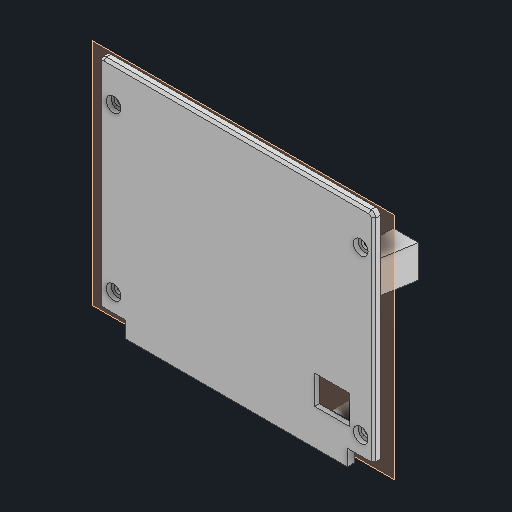
# Autodesk Inventor part: BP_BackCover
Saved by Autodesk Inventor 2026.1 (Build 301233020, 233B)
## iProperties
Created: 2025-09-13
Part Number: BP_BackCover
Material: Generic
Document SubType Name: Modeling
Designer: atrus
Density: 1 g/cm^3
Appearance: Default
Author: atrus
Autodesk Inventor part; units mm, degrees
ref_plane "YZ Plane" through (0, 0, 0) normal (1, 0, 0) x (0, 1, 0)
ref_plane "XZ Plane" through (0, 0, 0) normal (0, 1, 0) x (-1, 0, 0)
ref_plane "XY Plane" through (0, 0, 0) normal (0, 0, 1) x (1, 0, 0)
ref_plane "Work Plane1" through (0, 0, -0.1) normal (0, 0, 1) x (1, 0, 0)
sketch "Sketch1" plane through (0, 0, -0.1) normal (0, 0, 1) x (1, 0, 0)
  circle A0 centre (-111.199, -72) radius 2
  circle A1 centre (-5.483, -2.5) radius 2
  circle A2 centre (-111.199, -2.5) radius 2
  line L0 (-105.066, 0.2) -> (-96.966, 0.2)
  line L1 (-10.366, -5.012) -> (0, -5.012)
  line L2 (0, -5.012) -> (0, 5.5)
  line L3 (-9, 5.5) -> (0, 5.5)
  line L4 (-9, 5.5) -> (-9, 7.2)
  spline S0 degree 3 poles (-11.0328, 9.2) (-10.764, 9.2) (-10.4976, 9.1476) (-10.0026, 8.9441) (-9.7782, 8.7957) (-9.4033, 8.4236) (-9.2552, 8.2048) (-9.0524, 7.7216) (-9, 7.4622) (-9, 7.2) knots 0 0 0 0 0.253656 0.253656 0.505123 0.505123 0.752333 0.752333 1 1 1 1
  line L5 (-106.2992, 9.2) -> (-11.0328, 9.2)
  spline S1 degree 3 poles (-108.332, 7.2) (-108.332, 7.4565) (-108.2819, 7.7103) (-108.0866, 8.187) (-107.9426, 8.4048) (-107.577, 8.7772) (-107.3577, 8.9271) (-106.9875, 9.0869) (-106.8536, 9.1291) (-106.5792, 9.1857) (-106.4394, 9.2) (-106.2992, 9.2) knots 0 0 0 0 0.242386 0.242386 0.486827 0.486827 0.735395 0.735395 0.867613 0.867613 1 1 1 1
  line L6 (-108.332, 5.5) -> (-108.332, 7.2)
  line L7 (-117.332, 5.5) -> (-108.332, 5.5)
  line L8 (-117.332, -80) -> (-117.332, 5.5)
  line L9 (-105.066, -80) -> (-117.332, -80)
  line L10 (-105.066, -80) -> (-105.066, 0.2)
  circle A3 centre (-5.483, -72) radius 2
  line L11 (0, -19.352) -> (-10.366, -19.352)
  line L12 (-10.966, -79.0494) -> (-10.966, -80)
  line L13 (0, -80) -> (-10.966, -80)
  line L14 (0, -19.352) -> (0, -80)
  line L15 (0, -19.352) -> (0, -5.012)
  line L16 (-10.366, 2) -> (-10.366, -5.012)
  line L17 (-96.966, 0.2) -> (-96.966, 2)
  arc A4 (-93.166, 5.8) -> (-96.966, 2) centre (-93.166, 2) ccw
  line L18 (-93.166, 5.8) -> (-14.166, 5.8)
  arc A5 (-10.366, 2) -> (-14.166, 5.8) centre (-14.166, 2) ccw
  line L19 (-10.366, -19.352) -> (-10.366, -77)
  arc A6 (-10.966, -79.0494) -> (-10.366, -77) centre (-14.166, -77) ccw
  line L20 (-10.366, -19.352) -> (-10.366, -5.012)
  line L21 (-105.066, -80) -> (-104.866, -80)
  line L22 (-106.132, -86.7) -> (-11.166, -86.7)
  line L23 (-11.166, -86.7) -> (-11.166, -80)
  line L24 (-11.166, -80) -> (-10.966, -80)
  line L25 (-10.366, -73) -> (-105.066, -73)
  circle A7 centre (-111.199, -72) radius 2
  circle A8 centre (-5.483, -2.5) radius 2
  circle A9 centre (-111.199, -2.5) radius 2
  line L26 (-10.366, 2) -> (-10.366, -5.012)
  line L27 (-10.366, -5.012) -> (0, -5.012)
  line L28 (0, -5.012) -> (0, 10.6)
  spline S2 degree 3 poles (-2.0424, 12.6) (-1.7711, 12.6) (-1.5022, 12.5471) (-1.0034, 12.3419) (-0.7775, 12.1926) (-0.4014, 11.8187) (-0.2533, 11.5995) (-0.0519, 11.1175) (0, 10.8602) (0, 10.6) knots 0 0 0 0 0.255338 0.255338 0.507826 0.507826 0.754805 0.754805 1 1 1 1
  line L29 (-115.2896, 12.6) -> (-2.0424, 12.6)
  spline S3 degree 3 poles (-117.332, 10.6) (-117.332, 10.8554) (-117.2821, 11.108) (-117.0875, 11.5833) (-116.9438, 11.8006) (-116.5783, 12.1734) (-116.3584, 12.3239) (-115.9863, 12.4852) (-115.8508, 12.528) (-115.5731, 12.5855) (-115.4315, 12.6) (-115.2896, 12.6) knots 0 0 0 0 0.240766 0.240766 0.484156 0.484156 0.732838 0.732838 0.866308 0.866308 1 1 1 1
  line L30 (-117.332, -80) -> (-117.332, 10.6)
  line L31 (-105.066, -80) -> (-117.332, -80)
  line L32 (-105.066, -80) -> (-105.066, 3.6)
  line L33 (-105.066, 3.6) -> (-96.6127, 3.6)
  arc A10 (-93.166, 5.8) -> (-96.6127, 3.6) centre (-93.166, 2) ccw
  line L34 (-93.166, 5.8) -> (-14.166, 5.8)
  arc A11 (-10.366, 2) -> (-14.166, 5.8) centre (-14.166, 2) ccw
  line L35 (-106.132, -86.9) -> (-106.132, -97.8) construction
  line L36 (-106.132, -86.7) -> (-106.132, -80)
  line L37 (-117.332, -79.8) -> (-105.066, -79.8)
  line L38 (-10.966, -79.8) -> (0, -79.8)
  line L39 (-106.132, -80) -> (-106.132, -79.8)
  point P0 (0, 0)
  dimension "d1" = 0.2
  dimension "d3" = 7
  dimension "d36" = 0.2
  dimension "d37" = 0.2
  constraints: 22 end point, 12 point on line, 4 perpendicular, 2 horizontal, 2 vertical
  measures "d1" distance from line of L12.end L23
  measures "d3" distance from line of L23.end L25
  measures "d36" distance between parallel lines of L13 L38
  measures "d37" distance of L22.start L35.start
extrude "Extrusion1" add sketch "Sketch1" along normal blind 1.8 contours A0 | A1 | A2 | L32 L33 A4 L17 L0 | L10 L37 L8 L7 L6 S1 L5 S0 L4 L3 L2 L1 L16 A5 L18 A4 L33 L32 | L25 L19 A6 L12 L24 L23 L22 L36 L9 L10 | L10 L9 L39 L37 | L19 L11 L14 L38 L12 A6 | L20 L1 L15 L11 | L30 S3 L29 S2 L28 L3 L4 S0 L5 S1 L6 L7 | A3
sketch "Sketch2" plane through (0, 0, 1.7) normal (0, 0, 1) x (1, 0, 0)
  line L0 (-106.132, -86.7) -> (-11.166, -86.7) projected
  line L1 (-11.166, -86.7) -> (-11.166, -80) projected
  line L2 (-10.366, 2) -> (-10.366, -73) projected
  line L3 (-10.366, -73) -> (-105.066, -73) projected
  line L4 (-105.066, -73) -> (-105.066, 0.2) projected
  line L5 (-105.066, 0.2) -> (-96.966, 0.2) projected
  line L6 (-96.966, 0.2) -> (-96.966, 2) projected
  arc A0 (-93.166, 5.8) -> (-96.966, 2) centre (-93.166, 2) ccw projected
  line L7 (-93.166, 5.8) -> (-14.166, 5.8) projected
  arc A1 (-10.366, 2) -> (-14.166, 5.8) centre (-14.166, 2) ccw projected
  line L8 (-11.166, -86.9) -> (-106.132, -86.9) projected
  line L9 (-11.166, -86.7) -> (-104.866, -86.7)
  line L10 (-117.332, -79.8) -> (-106.132, -79.8) projected
  line L11 (-11.166, -80) -> (-10.966, -80) projected
  line L12 (-10.966, -80) -> (-10.966, -79.8) projected
  line L13 (-10.966, -79.8) -> (0, -79.8) projected
  line L14 (0, -79.8) -> (0, 10.6) projected
  line L15 (-106.132, -79.8) -> (-106.132, -86.7) projected
  ellipse E0 centre (-2.0424, 10.6) end of major axis (0, 10.6) minor radius 2 (0, 10.6) -> (-2.0424, 12.6) ccw projected
  line L16 (-2.0424, 12.6) -> (-115.2896, 12.6) projected
  ellipse E1 centre (-115.2896, 10.6) end of major axis (-113.2473, 10.5998) minor radius 2 (-115.2896, 12.6) -> (-117.332, 10.6) ccw projected
  line L17 (-117.332, 10.6) -> (-117.332, -79.8) projected
  point P0 (0, 0)
  dimension "d35" = 0.2
  constraints: 2 end point, 1 parallel, 1 point on line, 2 other
  measures "d35" distance between parallel lines of L8 L9
extrude "Extrusion2" add sketch "Sketch2" along normal blind 1.2 contours L15 L10 L17 E1 L16 E0 L14 L13 L12 L11 L1 L0 | L2 L3 L4 L5 L6 A0 L7 A1
sketch "Sketch3" plane through (0, 0, 2.9) normal (0, 0, 1) x (1, 0, 0)
  line L0 (-11.166, -71) -> (-24.166, -71) projected
  line L1 (-11.166, -60) -> (-11.166, -71) projected
  line L2 (-24.166, -60) -> (-11.166, -60) projected
  line L3 (-24.166, -71) -> (-24.166, -60) projected
  line L4 (-24.166, -70.3) -> (-11.166, -70.3)
  point P0 (0, 0)
  dimension "d34" = 0.7
  constraints: 2 end point, 2 point on line, 1 horizontal
  measures "d34" distance between parallel lines of L0 L4
extrude "Extrusion3" cut sketch "Sketch3" against normal blind 3 contours L4 L3 L2 L1
sketch "Sketch4" plane through (0, 0, 2.9) normal (0, 0, 1) x (1, 0, 0)
  circle A0 centre (-5.483, -2.5) radius 2 construction
  circle A1 centre (-5.483, -72) radius 2 construction
  circle A2 centre (-111.199, -2.5) radius 2 construction
  circle A3 centre (-111.199, -72) radius 2 construction
  point P0 (0, 0)
  constraints: 4 coincident
hole "Hole1" at (-111.199, -72, 2.9) at (-111.199, -2.5, 2.9) at (-5.483, -2.5, 2.9) at (-5.483, -72, 2.9) direction (0, 0, -1) diameter 3.4 end through all counterbore diameter 6.3 counterbore depth 2 clearance for "Flat Head Machine Screw" size "M3" standard "Ansi Metric M Profile"
chamfer "Chamfer1" distance 1 angle 45 4 edges at (-24.166, -65.15, 2.9) (-17.666, -60, 2.9) (-11.166, -65.15, 2.9) (-17.666, -70.3, 2.9)
sketch "Sketch5" plane through (0, 0, -0.1) normal (0, 0, -1) x (-1, 0, 0)
  line L0 (0, -19.352) -> (10.366, -19.352) projected
  line L1 (0, -79.8) -> (0, 10.6) projected
  line L2 (10.366, 2) -> (10.366, -73) projected
  line L3 (10.366, -5.012) -> (0, -5.012) projected
  line L4 (0, -19.152) -> (10.366, -19.152)
  line L5 (0, -5.212) -> (10.366, -5.212)
  point P0 (0, 0)
  point P1 (0, -80)
  point P2 (0, 5.5)
  dimension "d20" = 0.2
  dimension "d21" = 0.2
  constraints: 4 end point, 2 perpendicular, 2 point on line, 3 other
  measures "d20" distance between parallel lines of L3 L5
  measures "d21" distance between parallel lines of L0 L4
extrude "Extrusion4" add sketch "Sketch5" along normal blind 8 contours L1 L5 L2 L4
sketch "Sketch7" plane through (-10.366, -5.212, -0.1) normal (0, 1, 0) x (1, 0, 0)
  line L0 (10.366, -0.1) -> (10.366, 8) projected
  line L1 (0, 13.9798) -> (12.7429, 13.9798) projected
  line L2 (0, 8) -> (10.366, 8) projected
  line L3 (0, 0) -> (0, 13.6) projected
  line L4 (2, 13.9798) -> (2, 8)
  line L5 (2, 13.7798) -> (12.7859, 13.7798)
  spline S0 degree 3 poles (1.366, 54.07) (2.6114, 54.07) (3.9309, 53.8595) (6.2483, 52.8955) (7.2365, 52.2155) (8.6015, 50.9016) (9.0798, 50.326) (10.3635, 48.5092) (10.9891, 47.2127) (11.8316, 45.0211) (12.1129, 44.127) (12.7735, 41.6602) (13.0681, 40.0838) (13.5276, 36.7721) (13.6742, 35.0374) (13.8523, 31.3701) (13.8669, 29.4389) (13.7666, 24.7854) (13.5948, 22.0679) (13.041, 16.0946) (12.6224, 12.8476) (11.6152, 6.396) (11.0258, 3.1892) (10.366, 0) knots 0 0 0 0 0.309903 0.309903 0.584179 0.584179 0.77016 0.77016 1.152617 1.152617 1.413042 1.413042 1.86998 1.86998 2.374169 2.374169 2.940222 2.940222 3.743245 3.743245 4.712988 4.712988 5.681003 5.681003 5.681003 5.681003 projected
  point P0 (12.7169, 13.7798)
  point P1 (10.366, 0)
  dimension "d24" = 0.2
  dimension "d25" = 2
  constraints: 4 end point, 3 point on line, 1 perpendicular, 1 vertical
  measures "d24" distance between parallel lines of L1 L5
  measures "d25" distance between parallel lines of L3 L4
extrude "Extrusion5" add sketch "Sketch7" against normal up to surface (13.94 mm away) contours L0 L2 L4 L5 S0
sketch "Sketch8" plane through (0, 0, 1.7) normal (0, 0, -1) x (-1, 0, 0)
  circle A0 centre (17.916, -73.25) radius 1.8 projected
  circle A1 centre (17.916, -73.25) radius 1.8 projected
  circle A2 centre (17.916, -1.75) radius 1.8 projected
  circle A3 centre (89.416, -1.75) radius 1.8 projected
  circle A4 centre (89.416, -73.25) radius 1.8 projected
  circle A5 centre (89.416, -1.75) radius 2.8
  circle A6 centre (17.916, -1.75) radius 2.8
  circle A7 centre (17.916, -73.25) radius 2.8
  circle A8 centre (89.416, -73.25) radius 2.8
  point P0 (0, 0)
  dimension "d28" = 1
  dimension "d29" = 1
  dimension "d30" = 1
  dimension "d31" = 1
  constraints: 4 centre point, 2 coincident
  measures "d28" radial gap between concentric circles of A8 A4
  measures "d29" radial gap between concentric circles of A7 A0
  measures "d30" radial gap between concentric circles of A6 A2
  measures "d31" radial gap between concentric circles of A5 A3
ref_plane "Work Plane2" through (-96.166, -80, -11.9798) normal (0, 0, 1) x (1, 0, 0)
extrude "Extrusion6" add sketch "Sketch8" along normal up to surface (13.6798 mm away)
chamfer "Chamfer2" distance 1 angle 45 1 edges at (0, -34.6, 2.9)
body "Solid1"
